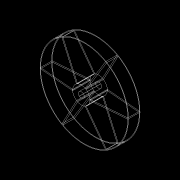
# Autodesk Inventor part: Wheel_Spokes
Saved by Autodesk Inventor 2011 SP1 (Build 150282100, 282)
## iProperties
Created: 2013-01-14
Part Number: Wheel_Spokes
Document SubType Name: Modeling
Designer: 939551
Density: 1 g/cm^3
Author: 939551
Autodesk Inventor part; units mm, degrees
ref_plane "YZ Plane" through (0, 0, 0) normal (1, 0, 0) x (0, 1, 0)
ref_plane "XZ Plane" through (0, 0, 0) normal (0, 1, 0) x (-1, 0, 0)
ref_plane "XY Plane" through (0, 0, 0) normal (0, 0, 1) x (1, 0, 0)
sketch "Sketch1" plane through (0, 0, 0) normal (0, 0, 1) x (1, 0, 0)
  circle A0 centre (0, 0) radius 97.155
  circle A1 centre (0, 0) radius 95.885
  dimension "d0" = 194.31
  dimension "d1" = 191.77
  constraints: 2 centre point, 2 coincident
  measures "d0" diameter of A0
  measures "d1" diameter of A1
extrude "Extrusion1" add sketch "Sketch1" along normal mid plane 25.4
sketch "Sketch2" plane through (0, 0, 0) normal (0, 0, 1) x (1, 0, 0)
  circle A0 centre (0, 0) radius 19.05
  circle A1 centre (0, 0) radius 6.35
  dimension "d4" = 38.1
  dimension "d5" = 12.7
  constraints: 2 centre point, 2 coincident
  measures "d4" diameter of A0
  measures "d5" diameter of A1
extrude "Extrusion2" add sketch "Sketch2" along normal mid plane 38.1
sketch "Sketch3" plane through (0, 0, 0) normal (0, 1, 0) x (-1, 0, 0)
  line L0 (95.885, -12.7) -> (-95.885, -12.7) projected
  line L1 (-95.885, 12.7) -> (95.885, 12.7) projected
  line L2 (19.05, -19.05) -> (19.05, 19.05) projected
  line L3 (19.05, 19.05) -> (19.05, -19.05)
  line L4 (19.05, -19.05) -> (95.885, -12.7)
  line L5 (95.885, -12.7) -> (95.885, 12.7)
  line L6 (95.885, 12.7) -> (19.05, 19.05)
  constraints: 8 end point, 1 collinear, 1 parallel
extrude "Extrusion3" add sketch "Sketch3" along normal mid plane 2.54
pattern_circular "Circular Pattern1" count 6 over 360 about axis through (0, 0, 19.05) along (0, 0, -1) of "Extrusion3"
body "Solid1"
